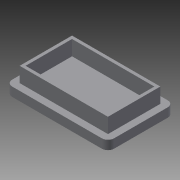
# Autodesk Inventor part: Tapa
Saved by Autodesk Inventor 2013 (Build 170138000, 138)
## iProperties
Created: 2014-07-03
Part Number: Tapa
Material: Genérico
Document SubType Name: Chapa
Designer: Administrador
Density: 1 g/cm^3
Sheet Metal Rule: Por defecto_mm
Author: Administrador
Autodesk Inventor part; units mm, degrees
note: some values were not read from the file. Chosen so that the rebuilt part matches the saved one: direction of "Repujado1".
ref_plane "YZ Plane" through (0, 0, 0) normal (1, 0, 0) x (0, 1, 0)
ref_plane "XZ Plane" through (0, 0, 0) normal (0, 1, 0) x (-1, 0, 0)
ref_plane "XY Plane" through (0, 0, 0) normal (0, 0, 1) x (1, 0, 0)
sketch "Boceto1" plane through (0, 0, 0) normal (0, 0, 1) x (1, 0, 0)
  line L0 (-7.2671, 8.5953) -> (26.7329, 8.5953)
  line L1 (26.7329, 8.5953) -> (26.7329, -13.4047)
  line L2 (26.7329, -13.4047) -> (-7.2671, -13.4047)
  line L3 (-7.2671, -13.4047) -> (-7.2671, 8.5953)
  point P0 (0, 0)
  dimension "d0" = 34
  dimension "d1" = 22
  constraints: 8 end point, 2 parallel, 1 horizontal, 1 perpendicular
  measures "d0" distance of L1.end L2.end
  measures "d1" distance of L0.end L1.end
extrude "Extrusión1" add sketch "Boceto1" along normal blind 3
sketch "Boceto2" plane through (0, 0, 3) normal (0, 0, 1) x (1, 0, 0)
  line L0 (-7.2671, 8.5953) -> (26.7329, -13.4047) construction
  line L1 (26.7329, 8.5953) -> (-7.2671, -13.4047) construction
  line L2 (-5.0171, 6.3453) -> (24.4829, 6.3453)
  line L3 (24.4829, 6.3453) -> (24.4829, -11.1547)
  line L4 (24.4829, -11.1547) -> (-5.0171, -11.1547)
  line L5 (-5.0171, -11.1547) -> (-5.0171, 6.3453)
  line L6 (-5.0171, 6.3453) -> (24.4829, -11.1547) construction
  line L7 (-5.0171, -11.1547) -> (24.4829, 6.3453) construction
  line L8 (-4.0171, 5.3453) -> (23.4829, 5.3453)
  line L9 (23.4829, 5.3453) -> (23.4829, -10.1547)
  line L10 (23.4829, -10.1547) -> (-4.0171, -10.1547)
  line L11 (-4.0171, -10.1547) -> (-4.0171, 5.3453)
  line L12 (-4.0171, 5.3453) -> (23.4829, -10.1547) construction
  line L13 (23.4829, 5.3453) -> (-4.0171, -10.1547) construction
  point P0 (0, 0)
  point P1 (9.7329, -2.4047)
  dimension "d4" = 29.5
  dimension "d5" = 17.5
  dimension "d6" = 27.5
  dimension "d7" = 15.5
  constraints: 28 end point, 4 parallel, 3 midpoint, 2 horizontal, 2 perpendicular
  measures "d4" distance of L3.end L4.end
  measures "d5" distance of L2.end L3.end
  measures "d6" distance of L9.end L10.end
  measures "d7" distance of L8.end L9.end
extrude "Extrusión2" add sketch "Boceto2" along normal blind 5
fillet "Empalme1" radius 2 4 edges at (26.7329, 8.5953, 1.5) (-7.2671, 8.5953, 1.5) (26.7329, -13.4047, 1.5) (-7.2671, -13.4047, 1.5)
sketch "Boceto4" plane through (0, 0, 0) normal (0, 0, -1) x (-1, 0, 0)
  line L0 (-23.6859, 1.5715) -> (4.87, 1.5715) construction
  line L1 (4.87, 1.5715) -> (4.87, -9.0557) construction
  line L2 (4.87, -9.0557) -> (-23.6859, -9.0557) construction
  line L3 (-23.6859, -9.0557) -> (-23.6859, 1.5715) construction
  line L4 (-23.1142, -4.696) -> (-23.1142, 1.304)
  line L5 (-23.1142, 1.304) -> (-21.9023, 1.304)
  line L6 (-21.9023, 1.304) -> (-21.9023, -4.696)
  line L7 (-21.9023, -4.696) -> (-23.1142, -4.696)
  line L8 (-15.4165, -4.696) -> (-15.4165, -2.435)
  spline S0 degree 2 poles (-15.4165, -2.435) (-15.4165, -2.0995) (-15.4408, -1.6425) (-15.4991, -1.4966) knots 0 0 0 1 2 2 2
  spline S1 degree 2 poles (-15.4991, -1.4966) (-15.5623, -1.3508) (-15.8152, -1.2195) (-16.0437, -1.2195) knots 0 0 0 1 2 2 2
  spline S2 degree 2 poles (-16.0437, -1.2195) (-16.2041, -1.2195) (-16.5153, -1.3605) (-16.7001, -1.4918) knots 0 0 0 1 2 2 2
  line L9 (-16.7001, -1.4918) -> (-16.7001, -4.696)
  line L10 (-16.7001, -4.696) -> (-18.1199, -4.696)
  line L11 (-18.1199, -4.696) -> (-18.1199, -2.435)
  spline S3 degree 2 poles (-18.1199, -2.435) (-18.1199, -2.1044) (-18.149, -1.6425) (-18.2074, -1.4966) knots 0 0 0 1 2 2 2
  spline S4 degree 2 poles (-18.2074, -1.4966) (-18.2706, -1.3508) (-18.5234, -1.2195) (-18.752, -1.2195) knots 0 0 0 1 2 2 2
  spline S5 degree 2 poles (-18.752, -1.2195) (-18.9221, -1.2195) (-19.2576, -1.3799) (-19.4132, -1.4918) knots 0 0 0 1 2 2 2
  line L12 (-19.4132, -1.4918) -> (-19.4132, -4.696)
  line L13 (-19.4132, -4.696) -> (-20.8233, -4.696)
  line L14 (-20.8233, -4.696) -> (-20.8233, -0.1692)
  line L15 (-20.8233, -0.1692) -> (-19.4132, -0.1692)
  line L16 (-19.4132, -0.1692) -> (-19.4132, -0.67)
  spline S6 degree 2 poles (-19.4132, -0.67) (-19.068, -0.3783) (-18.4505, -0.0477) (-18.0664, -0.0477) knots 0 0 0 1 2 2 2
  spline S7 degree 2 poles (-18.0664, -0.0477) (-17.6531, -0.0477) (-17.021, -0.4415) (-16.8557, -0.8354) knots 0 0 0 1 2 2 2
  spline S8 degree 2 poles (-16.8557, -0.8354) (-16.4521, -0.4561) (-15.7325, -0.0477) (-15.363, -0.0477) knots 0 0 0 1 2 2 2
  spline S9 degree 2 poles (-15.363, -0.0477) (-15.0469, -0.0477) (-14.5461, -0.247) (-14.3759, -0.4512) knots 0 0 0 1 2 2 2
  spline S10 degree 2 poles (-14.3759, -0.4512) (-14.1863, -0.67) (-13.9967, -1.2681) (-13.9967, -1.7495) knots 0 0 0 1 2 2 2
  line L17 (-13.9967, -1.7495) -> (-13.9967, -4.696)
  line L18 (-13.9967, -4.696) -> (-15.4165, -4.696)
  spline S11 degree 2 poles (-11.2203, -4.7835) (-12.081, -4.7835) (-12.8686, -4.0736) (-12.8686, -3.2665) knots 0 0 0 1 2 2 2
  line L19 (-12.8686, -3.2665) -> (-12.8686, -1.1514)
  line L20 (-12.8686, -1.1514) -> (-13.4084, -1.1514)
  line L21 (-13.4084, -1.1514) -> (-13.4084, -0.1692)
  line L22 (-13.4084, -0.1692) -> (-12.8686, -0.1692)
  line L23 (-12.8686, -0.1692) -> (-12.8686, 1.1241)
  line L24 (-12.8686, 1.1241) -> (-11.4586, 1.1241)
  line L25 (-11.4586, 1.1241) -> (-11.4586, -0.1692)
  line L26 (-11.4586, -0.1692) -> (-10.0972, -0.1692)
  line L27 (-10.0972, -0.1692) -> (-10.0972, -1.1514)
  line L28 (-10.0972, -1.1514) -> (-11.4586, -1.1514)
  line L29 (-11.4586, -1.1514) -> (-11.4586, -2.7608)
  spline S12 degree 2 poles (-11.4586, -2.7608) (-11.4586, -2.9991) (-11.4489, -3.354) (-11.3905, -3.495) knots 0 0 0 1 2 2 2
  spline S13 degree 2 poles (-11.3905, -3.495) (-11.3322, -3.636) (-11.0453, -3.8013) (-10.773, -3.8013) knots 0 0 0 1 2 2 2
  spline S14 degree 2 poles (-10.773, -3.8013) (-10.6563, -3.8013) (-10.2917, -3.7041) (-10.2187, -3.6652) knots 0 0 0 1 2 2 2
  line L30 (-10.2187, -3.6652) -> (-10.0972, -3.6652)
  line L31 (-10.0972, -3.6652) -> (-10.0972, -4.6571)
  spline S15 degree 2 poles (-10.0972, -4.6571) (-10.3257, -4.7154) (-10.8411, -4.7835) (-11.2203, -4.7835) knots 0 0 0 1 2 2 2
  spline S16 degree 2 poles (-7.2041, -4.8175) (-8.4878, -4.8175) (-9.8541, -3.5922) (-9.8541, -2.4593) knots 0 0 0 1 2 2 2
  spline S17 degree 2 poles (-9.8541, -2.4593) (-9.8541, -1.3508) (-8.5802, -0.0282) (-7.4327, -0.0282) knots 0 0 0 1 2 2 2
  spline S18 degree 2 poles (-7.4327, -0.0282) (-6.397, -0.0282) (-5.3468, -1.1514) (-5.3468, -2.1919) knots 0 0 0 1 2 2 2
  line L32 (-5.3468, -2.1919) -> (-5.3468, -2.7025)
  line L33 (-5.3468, -2.7025) -> (-8.444, -2.7025)
  spline S19 degree 2 poles (-8.444, -2.7025) (-8.4246, -3.0185) (-8.196, -3.4367) (-8.0113, -3.5631) knots 0 0 0 1 2 2 2
  spline S20 degree 2 poles (-8.0113, -3.5631) (-7.8314, -3.6895) (-7.3451, -3.7965) (-7.0583, -3.7965) knots 0 0 0 1 2 2 2
  spline S21 degree 2 poles (-7.0583, -3.7965) (-6.8152, -3.7965) (-6.3387, -3.6895) (-6.1393, -3.5971) knots 0 0 0 1 2 2 2
  spline S22 degree 2 poles (-6.1393, -3.5971) (-5.9643, -3.5242) (-5.6725, -3.3443) (-5.5802, -3.2762) knots 0 0 0 1 2 2 2
  line L34 (-5.5802, -3.2762) -> (-5.4294, -3.2762)
  line L35 (-5.4294, -3.2762) -> (-5.4294, -4.4431)
  spline S23 degree 2 poles (-5.4294, -4.4431) (-5.6045, -4.5112) (-5.8865, -4.6279) (-6.1393, -4.6862) knots 0 0 0 1 2 2 2
  spline S24 degree 2 poles (-6.1393, -4.6862) (-6.3678, -4.7495) (-6.8541, -4.8175) (-7.2041, -4.8175) knots 0 0 0 1 2 2 2
  spline S25 degree 2 poles (-6.7374, -1.8516) (-6.7471, -1.4042) (-7.1409, -0.9326) (-7.5445, -0.9326) knots 0 0 0 1 2 2 2
  spline S26 degree 2 poles (-7.5445, -0.9326) (-7.9578, -0.9326) (-8.4246, -1.4285) (-8.4489, -1.8516) knots 0 0 0 1 2 2 2
  line L36 (-8.4489, -1.8516) -> (-6.7374, -1.8516)
  spline S27 degree 2 poles (-2.4051, -4.8175) (-2.9643, -4.8175) (-3.893, -4.5355) (-4.2382, -4.2438) knots 0 0 0 1 2 2 2
  spline S28 degree 2 poles (-4.2382, -4.2438) (-4.5737, -3.9472) (-4.9529, -3.0574) (-4.9529, -2.4545) knots 0 0 0 1 2 2 2
  spline S29 degree 2 poles (-4.9529, -2.4545) (-4.9529, -1.8029) (-4.5445, -0.8937) (-4.1896, -0.602) knots 0 0 0 1 2 2 2
  spline S30 degree 2 poles (-4.1896, -0.602) (-3.8541, -0.32) (-2.94, -0.0477) (-2.444, -0.0477) knots 0 0 0 1 2 2 2
  spline S31 degree 2 poles (-2.444, -0.0477) (-2.0696, -0.0477) (-1.3208, -0.2227) (-0.9416, -0.4123) knots 0 0 0 1 2 2 2
  line L37 (-0.9416, -0.4123) -> (-0.9416, -1.6182)
  line L38 (-0.9416, -1.6182) -> (-1.1215, -1.6182)
  spline S32 degree 2 poles (-1.1215, -1.6182) (-1.209, -1.5355) (-1.4521, -1.341) (-1.598, -1.2632) knots 0 0 0 1 2 2 2
  spline S33 degree 2 poles (-1.598, -1.2632) (-1.7536, -1.1757) (-2.1377, -1.059) (-2.3759, -1.059) knots 0 0 0 1 2 2 2
  spline S34 degree 2 poles (-2.3759, -1.059) (-2.9156, -1.059) (-3.5088, -1.8127) (-3.5088, -2.4545) knots 0 0 0 1 2 2 2
  spline S35 degree 2 poles (-3.5088, -2.4545) (-3.5088, -3.1352) (-2.8767, -3.8062) (-2.3516, -3.8062) knots 0 0 0 1 2 2 2
  spline S36 degree 2 poles (-2.3516, -3.8062) (-2.0842, -3.8062) (-1.6855, -3.6846) (-1.5396, -3.5971) knots 0 0 0 1 2 2 2
  spline S37 degree 2 poles (-1.5396, -3.5971) (-1.3986, -3.5144) (-1.1944, -3.3297) (-1.1215, -3.2568) knots 0 0 0 1 2 2 2
  line L39 (-1.1215, -3.2568) -> (-0.9416, -3.2568)
  line L40 (-0.9416, -3.2568) -> (-0.9416, -4.4674)
  spline S38 degree 2 poles (-0.9416, -4.4674) (-1.0631, -4.5209) (-1.3792, -4.6571) (-1.5445, -4.7008) knots 0 0 0 1 2 2 2
  spline S39 degree 2 poles (-1.5445, -4.7008) (-1.7487, -4.7592) (-2.1085, -4.8175) (-2.4051, -4.8175) knots 0 0 0 1 2 2 2
  line L41 (3.9644, -4.696) -> (2.5446, -4.696)
  line L42 (2.5446, -4.696) -> (2.5446, -2.4545)
  spline S40 degree 2 poles (2.5446, -2.4545) (2.5446, -2.1773) (2.5009, -1.6328) (2.4425, -1.5063) knots 0 0 0 1 2 2 2
  spline S41 degree 2 poles (2.4425, -1.5063) (2.3696, -1.3508) (2.0973, -1.2195) (1.8639, -1.2195) knots 0 0 0 1 2 2 2
  spline S42 degree 2 poles (1.8639, -1.2195) (1.6938, -1.2195) (1.3388, -1.3508) (1.1395, -1.4918) knots 0 0 0 1 2 2 2
  line L43 (1.1395, -1.4918) -> (1.1395, -4.696)
  line L44 (1.1395, -4.696) -> (-0.2706, -4.696)
  line L45 (-0.2706, -4.696) -> (-0.2706, 1.5715)
  line L46 (-0.2706, 1.5715) -> (1.1395, 1.5715)
  line L47 (1.1395, 1.5715) -> (1.1395, -0.67)
  spline S43 degree 2 poles (1.1395, -0.67) (1.4847, -0.3783) (2.1411, -0.0477) (2.5398, -0.0477) knots 0 0 0 1 2 2 2
  spline S44 degree 2 poles (2.5398, -0.0477) (3.2302, -0.0477) (3.9644, -0.9229) (3.9644, -1.7495) knots 0 0 0 1 2 2 2
  line L48 (3.9644, -1.7495) -> (3.9644, -4.696)
  point P0 (0, 0)
  constraints: 2 other
emboss "Repujado1" sketch "Boceto4" operation cut depth 0.5 direction (0, 0, 1)
equation "\"Radio_pliegue\" = Grosor"
equation "\"Anchura_desahogo_plegado\" = Grosor"
equation "\"Profundidad_desahogo_plegado\" = 0.5 * Grosor"
equation "\"Tamaño_destalonado\" = 4 * Grosor"
equation "\"Remanente_mínimo\" = 2 * Grosor"
equation "\"Radiodetransición\" = Radio_pliegue"
equation "\"Tamaño_de_radio_de_Jacobi\" = Radio_pliegue"
equation "\"TamañoSeparación\" = Grosor"
equation "\"Grosor\" = 0.5"
